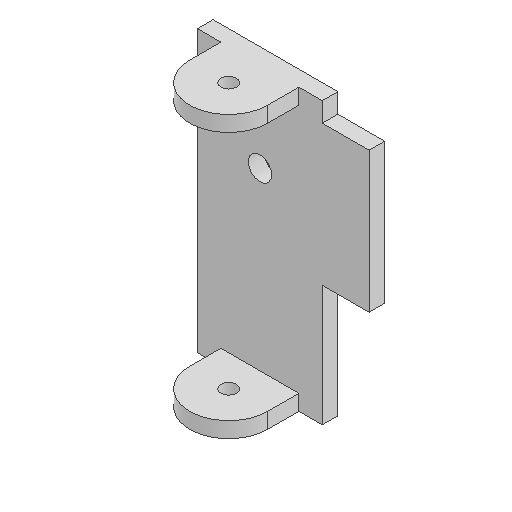
# Autodesk Inventor part: wheel_braket_front
Saved by Autodesk Inventor 2025.2 (Build 292293000, 293)
## iProperties
Created: 2024-02-12
Part Number: wheel_braket_front
Material: 일반
Document SubType Name: Modeling
Designer: ps737
Density: 1 g/cm^3
Appearance: 기본값
Author: ps737
Autodesk Inventor part; units mm, degrees
ref_plane "YZ Plane" through (0, 0, 0) normal (1, 0, 0) x (0, 1, 0)
ref_plane "XZ Plane" through (0, 0, 0) normal (0, 1, 0) x (-1, 0, 0)
ref_plane "XY Plane" through (0, 0, 0) normal (0, 0, 1) x (1, 0, 0)
sketch "스케치1" plane through (0, 0, 0) normal (0, 0, 1) x (1, 0, 0)
  line L0 (80, -122.5) -> (0, -122.5)
  line L1 (80, 45) -> (110, 45)
  line L2 (110, 45) -> (110, -45)
  line L3 (110, -45) -> (80, -45)
  line L4 (80, 57.5) -> (80, 45)
  line L5 (80, -45) -> (80, -122.5)
  line L6 (40, 57.5) -> (40, -122.5)
  circle A0 centre (40, 47.0427) radius 7.5
  circle A1 centre (-7.0427, 0) radius 7.5
  circle A2 centre (40, -47.0427) radius 7.5
  circle A3 centre (87.0427, 0) radius 7.5
  circle A4 centre (40, 0) radius 7.5
  line L7 (0, 57.5) -> (80, 57.5)
  line L8 (0, 0) -> (0, 57.5)
  line L9 (0, 0) -> (0, -122.5)
  dimension "d0" = 80
  dimension "d3" = 45
  dimension "d4" = 45
  dimension "d13" = 360
  dimension "d14" = 0
  dimension "d15" = 47.0427
  dimension "d16" = 47.0427
  dimension "d21" = 15
  dimension "d31" = 122.5
  dimension "d36" = 12.5
  dimension "d37" = 30
  constraints: 20 end point, 5 centre point, 5 perpendicular, 2 coincident, 2 midpoint, 1 horizontal, 1 vertical, 9 other
  measures "d0" distance of L0.start L0.end
  measures "d3" distance from line of point (0, 0) L1
  measures "d4" distance from line of point (0, 0) L3
  measures "d14" distance from line of L6 A0.centre
  measures "d15" vertical distance of point (0, 0) A0.centre
  measures "d16" vertical distance of L8.start A2.centre
  measures "d21" diameter of A4
  measures "d31" distance from line of L0 point (0, 0)
  measures "d36" distance between parallel lines of L1 L7
  measures "d37" distance between parallel lines of L2 L5
extrude "돌출1" add sketch "스케치1" against normal blind 10 contours L0 L6 A2 A4 A0 L7 L4 L1 L2 L3 L5 | L0 L9 A1 L8 L7 L6 A0 A4 A2 | A2 L6 | L6 A2 | L9 L8 A1 | A4 L6 | L6 A4 | A0 L6 | L6 A0 | A3 picked at (0.0843, 1.4393)
extrude "돌출3" cut sketch "스케치1" against normal blind 40 contours A4 L6 | L6 A4
sketch "스케치2" plane through (0, -122.5, 0) normal (0, -1, 0) x (1, 0, 0)
  line L0 (0, 0) -> (80, 0) projected
  line L1 (15, 0) -> (15, 20)
  line L2 (15, 20) -> (65, 20)
  line L3 (65, 20) -> (65, 0)
  arc A0 (65, 20) -> (15, 20) centre (40, 20) ccw
  circle A1 centre (40, 20) radius 5
  point P0 (40, 0)
  dimension "d24" = 20
  dimension "d25" = 50
  dimension "d26" = 25
  dimension "d28" = 10
  constraints: 6 end point, 2 centre point, 2 midpoint, 2 perpendicular, 2 point on circle, 2 point on line, 1 coincident, 1 vertical
  measures "d24" distance between parallel lines of L0 L2
  measures "d25" distance between parallel lines of L3 L1
  measures "d26" distance from line of point (40, 0) L1
  measures "d28" diameter of A1
extrude "돌출4" add sketch "스케치2" against normal blind 10 contours L1 L2 A1 L3 L0 | A0 L2 A1
sketch "스케치3" plane through (0, 57.5, 0) normal (0, 1, 0) x (1, 0, 0)
  line L0 (15, 0) -> (15, -20) projected
  line L1 (65, -20) -> (65, 0) projected
  arc A0 (15, -20) -> (65, -20) centre (40, -20) ccw projected
  circle A1 centre (40, -20) radius 5 projected
  line L2 (80, 0) -> (0, 0) projected
extrude "돌출5" add sketch "스케치3" against normal blind 10
